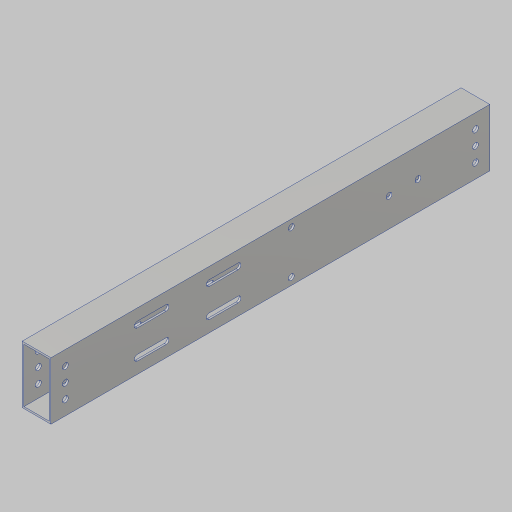
# Autodesk Inventor part: CL7-001
Saved by Autodesk Inventor 2023.5 (Build 275446000, 446)
## iProperties
RuleStatus: InUse
Created: 2025-03-17
Part Number: CL7-001
Material: Aluminum 6061
Document SubType Name: Modeling
Designer: dlangdon
Mass: 235.58 g
Surface Area: 1117.46 cm^2
Volume: 87.2519 cm^3
Density: 2.7 g/cm^3
Appearance: Aluminum - Flat
AfterDocNew0: SHOW
AfterDocOpen0: SHOW
Author: dlangdon
Autodesk Inventor part; units mm, degrees
ref_plane "YZ Plane" through (0, 0, 0) normal (1, 0, 0) x (0, 1, 0)
ref_plane "XZ Plane" through (0, 0, 0) normal (0, 1, 0) x (-1, 0, 0)
ref_plane "XY Plane" through (0, 0, 0) normal (0, 0, 1) x (1, 0, 0)
sketch "Sketch1" plane through (0, 0, 0) normal (0, 0, 1) x (1, 0, 0)
  line L0 (-12.7, -25.4) -> (12.7, -25.4)
  line L1 (12.7, -25.4) -> (12.7, 25.4)
  line L2 (12.7, 25.4) -> (-12.7, 25.4)
  line L3 (-12.7, 25.4) -> (-12.7, -25.4)
  line L4 (-12.7, -25.4) -> (12.7, 25.4) construction
  line L5 (12.7, -25.4) -> (-12.7, 25.4) construction
  line L6 (-11.1125, 23.8125) -> (11.1125, 23.8125)
  line L7 (11.1125, 23.8125) -> (11.1125, -23.8125)
  line L8 (11.1125, -23.8125) -> (-11.1125, -23.8125)
  line L9 (-11.1125, -23.8125) -> (-11.1125, 23.8125)
  point P0 (0, 0)
  dimension "width" = 25.4
  dimension "height" = 50.8
  dimension "thickness" = 1.5875
  constraints: 20 end point, 4 parallel, 2 midpoint, 2 perpendicular, 1 horizontal, 3 other
  measures "width" distance of L2.end L1.end
  measures "height" distance of L1.end L0.end
  measures "thickness" distance between parallel lines of L2 L6
extrude "Extrusion1" add sketch "Sketch1" along normal mid plane 387.35
sketch "Sketch2" plane through (12.7, -25.4, 193.675) normal (1, 0, 0) x (0, 0, -1)
  line L0 (387.35, 50.8) -> (387.35, 0) construction
  line L1 (387.35, 0) -> (0, 0) construction
  line L2 (0, 0) -> (0, 50.8) construction
  line L3 (0, 50.8) -> (387.35, 50.8) construction
  line L4 (387.35, 0) -> (0, 0) construction
  line L5 (0, 0) -> (0, 50.8) construction
  line L6 (0, 50.8) -> (387.35, 50.8) construction
  line L7 (387.35, 50.8) -> (387.35, 0) projected
  point P0 (193.675, 25.4)
  point P1 (12.7, 38.1)
  point P2 (12.7, 25.4)
  point P3 (0, 25.4)
  point P4 (12.7, 12.7)
  dimension "d5" = 12.7
  dimension "d6" = 12.7
  dimension "d7" = 12.7
  constraints: 2 vertical alignment, 1 horizontal alignment, 1 midpoint
  measures "d5" distance from line of L2 point (12.7, 25.4)
  measures "d6" distance of point (12.7, 25.4) point (12.7, 38.1)
  measures "d7" distance of point (12.7, 12.7) point (12.7, 25.4)
hole "Hole1" at (12.7, 12.7, 180.975) at (12.7, 0, 180.975) at (12.7, -12.7, 180.975) direction (-1, 0, 0) diameter 5.1054 end through all clearance for "Flat Head Machine Screw (82)" size "#10" standard "Ansi Unified Screw Threads"
mirror "Mirror1" about plane through (0, 0, 0) normal (0, 0, 1) of "Hole1"
sketch "Sketch3" plane through (12.7, -25.4, 193.675) normal (1, 0, 0) x (0, 0, -1)
  circle A0 centre (374.65, 12.7) radius 2.5527 construction
  circle A1 centre (374.65, 38.1) radius 2.5527 construction
  circle A2 centre (374.65, 25.4) radius 2.5527 construction
  circle A3 centre (12.7, 25.4) radius 2.5527 construction
  circle A4 centre (12.7, 38.1) radius 2.5527 construction
  circle A5 centre (12.7, 12.7) radius 2.5527 construction
  line L0 (387.35, 50.8) -> (387.35, 0) construction
  line L1 (387.35, 0) -> (0, 0) construction
  line L2 (0, 0) -> (0, 50.8) construction
  line L3 (0, 50.8) -> (387.35, 50.8) construction
  point P0 (193.675, 25.4)
  point P1 (323.85, 25.4)
  point P2 (298.45, 25.4)
  dimension "d15" = 50.8
  dimension "d16" = 25.4
  constraints: 2 horizontal alignment
  measures "d15" distance of point (323.85, 25.4) A2.centre
  measures "d16" distance of point (298.45, 25.4) point (323.85, 25.4)
hole "Hole2" at (12.7, 0, -130.175) at (12.7, 0, -104.775) direction (-1, 0, 0) diameter 5.1054 end through all clearance for "Flat Head Machine Screw (82)" size "#10" standard "Ansi Unified Screw Threads"
sketch "Sketch4" plane through (12.7, -25.4, 193.675) normal (1, 0, 0) x (0, 0, -1)
  line L0 (165.1, 38.1) -> (139.7, 38.1) construction
  line L1 (165.1, 40.6527) -> (139.7, 40.6527)
  line L2 (139.7, 35.5473) -> (165.1, 35.5473)
  arc A0 (165.1, 35.5473) -> (165.1, 40.6527) centre (165.1, 38.1) ccw
  arc A1 (139.7, 40.6527) -> (139.7, 35.5473) centre (139.7, 38.1) ccw
  line L3 (165.1, 12.7) -> (139.7, 12.7) construction
  line L4 (165.1, 15.2527) -> (139.7, 15.2527)
  line L5 (139.7, 10.1473) -> (165.1, 10.1473)
  arc A2 (165.1, 10.1473) -> (165.1, 15.2527) centre (165.1, 12.7) ccw
  arc A3 (139.7, 15.2527) -> (139.7, 10.1473) centre (139.7, 12.7) ccw
  line L6 (152.4, 38.1) -> (152.4, 12.7) construction
  line L7 (0, 0) -> (0, 50.8) construction
  line L8 (101.6, 38.1) -> (76.2, 38.1) construction
  line L9 (101.6, 40.6527) -> (76.2, 40.6527)
  line L10 (76.2, 35.5473) -> (101.6, 35.5473)
  arc A4 (101.6, 35.5473) -> (101.6, 40.6527) centre (101.6, 38.1) ccw
  arc A5 (76.2, 40.6527) -> (76.2, 35.5473) centre (76.2, 38.1) ccw
  line L11 (101.6, 12.7) -> (76.2, 12.7) construction
  line L12 (101.6, 15.2527) -> (76.2, 15.2527)
  line L13 (76.2, 10.1473) -> (101.6, 10.1473)
  arc A6 (101.6, 10.1473) -> (101.6, 15.2527) centre (101.6, 12.7) ccw
  arc A7 (76.2, 15.2527) -> (76.2, 10.1473) centre (76.2, 12.7) ccw
  line L14 (88.9, 38.1) -> (88.9, 12.7) construction
  point P0 (193.675, 25.4)
  point P1 (152.4, 25.4)
  point P2 (88.9, 25.4)
  dimension "d25" = 5.1054
  dimension "d26" = 25.4
  dimension "d27" = 25.4
  dimension "d28" = 152.4
  dimension "d29" = 5.1054
  dimension "d30" = 25.4
  dimension "d31" = 25.4
  dimension "d32" = 63.5
  constraints: 36 end point, 16 point on circle, 16 tangent, 8 centre point, 6 midpoint, 6 parallel, 6 vertical alignment, 2 equal radius, 2 horizontal, 2 horizontal alignment, 2 vertical
  measures "d25" diameter of A3
  measures "d26" distance of L0.start L0.end
  measures "d27" distance of L6.start L6.end
  measures "d28" distance between parallel lines of L7 L6
  measures "d29" diameter of A7
  measures "d30" distance of L8.start L8.end
  measures "d31" distance of L14.start L14.end
  measures "d32" distance between parallel lines of L6 L14
extrude "Extrusion2" cut sketch "Sketch4" against normal through all
sketch "Sketch5" plane through (12.7, -25.4, 193.675) normal (1, 0, 0) x (0, 0, -1)
  line L0 (212.1027, 44.45) -> (212.1027, 6.35) construction
  line L1 (387.35, 50.8) -> (387.35, 0) construction
  arc A0 (165.1, 35.5473) -> (165.1, 40.6527) centre (165.1, 38.1) ccw construction
  point P0 (193.675, 25.4)
  point P1 (212.1027, 25.4)
  point P2 (387.35, 25.4)
  point P3 (167.6527, 38.1)
  dimension "d35" = 38.1
  dimension "d36" = 44.45
  constraints: 2 end point, 2 midpoint, 1 horizontal alignment, 1 point on circle, 1 vertical, 1 vertical alignment
  measures "d35" distance of L0.start L0.end
  measures "d36" distance from line of L0 point (167.653, 38.1)
hole "Hole3" at (12.7, 19.05, -18.4277) at (12.7, -19.05, -18.4277) direction (-1, 0, 0) diameter 5.1054 end through all clearance for "Flat Head Machine Screw (82)" size "#10" standard "Ansi Unified Screw Threads"
equation "\"d7\" = d6"
body "Solid1"
